Autodesk Inventor part; units mm, degrees
(part 3 of 3)
sketch "Additional Alignment Holes Top" plane through (0, 0, 0) normal (0, 1, 0) x (1, 0, 0)
  circle A0 centre (-38.1, 76.2) radius 3.175 projected
  circle A1 centre (-33.096, 76.2) radius 1.0125 projected
  circle A2 centre (-43.104, 76.2) radius 1.0125 projected
  line L0 (-38.1, 76.2) -> (-38.1, 70.15)
  circle A3 centre (-38.1, 70.15) radius 3.175
  line L1 (-38.1, 70.15) -> (-33.096, 70.15)
  line L2 (-38.1, 70.15) -> (-43.104, 70.15)
  circle A4 centre (-43.104, 70.15) radius 1.0125
  circle A5 centre (-33.096, 70.15) radius 1.0125
  circle A6 centre (-329.6666, 527.8374) radius 3.175 projected
  line L3 (-329.6666, 527.8374) -> (-348.7166, 527.8374)
  circle A7 centre (-348.7166, 527.8374) radius 3.175
  circle A8 centre (-329.6666, 522.8334) radius 1.0125 projected
  circle A9 centre (-329.6666, 532.8414) radius 1.0125 projected
  line L4 (-348.7166, 527.8374) -> (-348.7166, 532.8414)
  line L5 (-348.7166, 527.8374) -> (-348.7166, 522.8334)
  circle A10 centre (-348.7166, 522.8334) radius 1.0125
  circle A11 centre (-348.7166, 532.8414) radius 1.0125
  circle A12 centre (-430.0666, 527.8374) radius 3.175 projected
  line L6 (-430.0666, 527.8374) -> (-404.6666, 527.8374)
  circle A13 centre (-404.6666, 527.8374) radius 3.175
  line L7 (-404.6666, 527.8374) -> (-404.6666, 532.8414)
  circle A14 centre (-404.6666, 522.8334) radius 1.0125
  circle A15 centre (-404.6666, 532.8414) radius 1.0125
  circle A16 centre (-266.1666, 527.8374) radius 3.175 projected
  line L8 (-266.1666, 527.8374) -> (-240.7666, 527.8374)
  circle A17 centre (-240.7666, 527.8374) radius 3.175
  circle A18 centre (-240.7666, 522.8334) radius 1.0125
  circle A19 centre (-240.7666, 532.8414) radius 1.0125
  line L9 (-240.7666, 527.8374) -> (-113.7666, 527.8374)
  circle A20 centre (-113.7666, 527.8374) radius 3.175
  circle A21 centre (-113.7666, 522.8334) radius 1.0125
  circle A22 centre (-113.7666, 532.8414) radius 1.0125
  line L10 (-348.7166, 527.8374) -> (-323.3166, 527.8374)
  line L11 (-323.3166, 527.8374) -> (-323.3166, 502.4374)
  line L12 (-323.3166, 527.8374) -> (-323.3166, 553.2374)
  line L13 (-323.3166, 553.2374) -> (-374.1166, 553.2374)
  line L14 (-374.1166, 553.2374) -> (-374.1166, 502.4374)
  point P0 (0, 0)
  dimension "d807" = 6.05
  dimension "d808" = 6.35
  dimension "d809" = 2.025
  dimension "d810" = 2.025
  dimension "d811" = 19.05
  dimension "d812" = 6.35
  dimension "d813" = 2.025
  dimension "d814" = 2.025
  dimension "d815" = 25.4
  dimension "d816" = 6.35
  dimension "d817" = 2.025
  dimension "d818" = 2.025
  dimension "d819" = 25.4
  dimension "d820" = 6.35
  dimension "d821" = 2.025
  dimension "d822" = 2.025
  dimension "d823" = 127
  dimension "d824" = 6.35
  dimension "d825" = 2.025
  dimension "d826" = 2.025
  dimension "d827" = 25.4
  dimension "d828" = 25.4
  dimension "d829" = 25.4
  dimension "d830" = 50.8
  dimension "d831" = 50.8
  constraints: 30 end point, 15 centre point, 12 coincident, 6 horizontal, 5 vertical, 3 perpendicular, 1 point on line
  measures "d807" distance of L0.start L0.end
  measures "d808" diameter of A3
  measures "d809" diameter of A4
  measures "d810" diameter of A5
  measures "d811" distance of L3.start L3.end
  measures "d812" diameter of A7
  measures "d813" diameter of A10
  measures "d814" diameter of A11
  measures "d815" distance of L6.start L6.end
  measures "d816" diameter of A13
  measures "d817" diameter of A14
  measures "d818" diameter of A15
  measures "d819" distance of L8.start L8.end
  measures "d820" diameter of A17
  measures "d821" diameter of A18
  measures "d822" diameter of A19
  measures "d823" distance of L9.start L9.end
  measures "d824" diameter of A20
  measures "d825" diameter of A21
  measures "d826" diameter of A22
  measures "d827" distance of L4.start L10.end
  measures "d828" distance of L10.end L11.end
  measures "d829" distance of L10.end L12.end
  measures "d830" distance of L12.end L13.end
  measures "d831" distance of L13.end L14.end
hole "Hole4" at (-323.3166, 0, -502.4374) at (-323.3166, 0, -553.2374) at (-374.1166, 0, -553.2374) at (-374.1166, 0, -502.4374) direction (0, -1, 0) diameter 4.9784 end through all thread size "1/4-20 UNC" class "2B" standard "ANSI Unified Screw Threads"
extrude "Extrusion23" cut sketch "Additional Alignment Holes Top" against normal blind 25.4 contours A3 L0 A0 | A0 L0 L2 A3 | A3 L1 L0 A0 | A0 L0 A3 | L2 L1 A3 | A7 L5 L3 | L3 L4 A7 | L5 A7 L4 | A13 L7 L6 | L6 L7 A13 | A17 L9 L8 | L8 L9 A17 | A20
extrude "Extrusion24" cut sketch "Additional Alignment Holes Top" against normal blind 4.445 contours A4 | A5 | A10 | A11 | A14 | A15 | A18 | A19 | A21 | A22
sketch "Sketch26" plane through (-323.3166, -12.7, 0) normal (0, -1, 0) x (1, 0, 0)
  arc A0 (287.8819, -71.8753) -> (282.5513, -71.8753) centre (285.2166, -70.15) ccw projected
  arc A1 (286.181, -73.175) -> (287.8819, -71.8753) centre (285.2166, -70.15) ccw projected
  circle A2 centre (285.2166, -70.15) radius 3.175 projected
  arc A3 (282.5513, -71.8753) -> (287.8819, -71.8753) centre (285.2166, -76.2) ccw projected
  circle A4 centre (285.2166, -70.15) radius 2.54
  circle A5 centre (285.2166, -12.7) radius 5.08 projected
  circle A6 centre (285.2166, -70.15) radius 5.08
  circle A7 centre (209.55, -527.8374) radius 3.175 projected
  circle A8 centre (82.55, -527.8374) radius 3.175 projected
  circle A9 centre (-25.4, -527.8374) radius 3.175 projected
  circle A10 centre (-81.35, -527.8374) radius 3.175 projected
  circle A11 centre (-81.35, -527.8374) radius 5.08
  circle A12 centre (-25.4, -527.8374) radius 5.08
  circle A13 centre (82.55, -527.8374) radius 5.08
  circle A14 centre (209.55, -527.8374) radius 5.08
  point P0 (323.3166, 0)
  dimension "d844" = 10.16
  dimension "d845" = 10.16
  dimension "d846" = 10.16
  dimension "d847" = 10.16
  dimension "d848" = 10.16
  constraints: 6 centre point, 6 coincident
  measures "d844" diameter of A6
  measures "d845" diameter of A11
  measures "d846" diameter of A12
  measures "d847" diameter of A13
  measures "d848" diameter of A14
extrude "Extrusion25" cut sketch "Sketch26" against normal blind 7.62 contours A1 A2 A0 | A3 A6 A2 A1 | A0 A3 A6 | A4 | A7 | A8 | A9 | A10 | A11 | A12 | A13 | A14
sketch "Sketch27" plane through (0, 0, 0) normal (0, 1, 0) x (1, 0, 0)
  arc A0 (-39.0644, 73.175) -> (-37.1356, 73.175) centre (-38.1, 70.15) ccw projected
  arc A1 (-37.1356, 73.175) -> (-39.0644, 73.175) centre (-38.1, 76.2) ccw projected
  line L0 (-38.1, 76.2) -> (-38.1, 63.5)
  circle A2 centre (-38.1, 63.5) radius 3.175
  line L1 (-38.1, 76.2) -> (-38.1, 88.9)
  circle A3 centre (-38.1, 88.9) radius 3.175
  line L2 (-38.1, 76.2) -> (-25.4, 76.2)
  line L3 (-38.1, 76.2) -> (-50.8, 76.2)
  circle A4 centre (-50.8, 76.2) radius 3.175
  circle A5 centre (-25.4, 76.2) radius 3.175
  line L4 (-38.1, 76.2) -> (-16.1, 76.2)
  line L5 (-38.1, 76.2) -> (-38.1, 98.2)
  line L6 (-38.1, 76.2) -> (-38.1, 54.2)
  circle A6 centre (-38.1, 98.2) radius 1.5125
  circle A7 centre (-38.1, 54.2) radius 1.5125
  point P0 (0, 0)
  dimension "d853" = 12.7
  dimension "d854" = 6.35
  dimension "d855" = 12.7
  dimension "d856" = 12.7
  dimension "d857" = 12.7
  dimension "d858" = 6.35
  dimension "d859" = 6.35
  dimension "d860" = 22
  dimension "d861" = 22
  dimension "d862" = 22
  dimension "d863" = 3.025
  dimension "d864" = 3.025
  constraints: 14 end point, 6 centre point, 6 coincident, 3 vertical, 2 horizontal, 1 point on line
  measures "d853" distance of L0.start L0.end
  measures "d854" diameter of A2
  measures "d855" distance of L0.start L1.end
  measures "d856" distance of L0.start L2.end
  measures "d857" distance of L0.start L3.end
  measures "d858" diameter of A4
  measures "d859" diameter of A5
  measures "d860" distance of L0.start L4.end
  measures "d861" distance of L0.start L5.end
  measures "d862" distance of L0.start L6.end
  measures "d863" diameter of A6
  measures "d864" diameter of A7
extrude "Extrusion26" cut sketch "Sketch27" against normal blind 25.4 contours A5 L4 L2 | L2 L4 A5 | A4
extrude "Extrusion27" cut sketch "Sketch27" against normal blind 4.445 contours A6 | A7
sketch "Sketch28" plane through (-323.3166, -12.7, 0) normal (0, -1, 0) x (1, 0, 0)
  circle A0 centre (297.9166, -76.2) radius 3.175 projected
  circle A1 centre (272.5166, -76.2) radius 3.175 projected
  circle A2 centre (297.9166, -76.2) radius 5.08
  circle A3 centre (272.5166, -76.2) radius 5.08
  point P0 (323.3166, 0)
  dimension "d869" = 10.16
  dimension "d870" = 10.16
  constraints: 2 centre point, 2 coincident
  measures "d869" diameter of A2
  measures "d870" diameter of A3
extrude "Extrusion28" cut sketch "Sketch28" against normal blind 7.62 contours A0 | A1 | A2 | A3
hole "Hole5" at (-38.1, 0, -88.9) at (-38.1, 0, -63.5) direction (0, -1, 0) diameter 4.9784 end through all thread size "1/4-20 UNC" class "2B" standard "ANSI Unified Screw Threads"
sketch "Sketch29" plane through (0, 0, 0) normal (0, 1, 0) x (1, 0, 0)
  circle A0 centre (-38.1, 63.5) radius 2.4892 projected
  circle A1 centre (-38.1, 88.9) radius 2.4892 projected
  circle A2 centre (-38.1, 98.2) radius 1.5125 projected
  circle A3 centre (-38.1, 54.2) radius 1.5125 projected
  circle A4 centre (-25.4, 76.2) radius 3.175 projected
  circle A5 centre (-50.8, 76.2) radius 3.175 projected
  circle A6 centre (-113.7666, 532.8414) radius 1.0125 projected
  circle A7 centre (-348.7166, 532.8414) radius 1.0125 projected
  circle A8 centre (-404.6666, 532.8414) radius 1.0125 projected
  circle A9 centre (-240.7666, 532.8414) radius 1.0125 projected
  circle A10 centre (-33.096, 70.15) radius 1.0125 projected
  circle A11 centre (-113.7666, 522.8334) radius 1.0125 projected
  circle A12 centre (-348.7166, 522.8334) radius 1.0125 projected
  circle A13 centre (-404.6666, 522.8334) radius 1.0125 projected
  circle A14 centre (-240.7666, 522.8334) radius 1.0125 projected
  circle A15 centre (-43.104, 70.15) radius 1.0125 projected
  circle A16 centre (-348.7166, 379.0684) radius 3.175 projected
  circle A17 centre (-348.7166, 127.6824) radius 3.175 projected
  circle A18 centre (-348.7166, -46.5176) radius 3.175 projected
  line L0 (-323.3166, 0) -> (0, 0) projected
  line L1 (0, 0) -> (0, 565.9374) projected
  line L2 (0, 565.9374) -> (-329.6666, 565.9374) projected
  line L3 (-329.6666, 565.9374) -> (-329.6666, 604.0374) projected
  line L4 (-329.6666, 604.0374) -> (-367.7666, 604.0374) projected
  line L5 (-367.7666, 604.0374) -> (-367.7666, 565.9374) projected
  line L6 (-367.7666, 565.9374) -> (-705.4595, 565.9374) projected
  line L7 (-705.4595, 565.9374) -> (-705.4595, 489.7374) projected
  line L8 (-705.4595, 489.7374) -> (-374.1166, 489.7374) projected
  line L9 (-374.1166, 489.7374) -> (-374.1166, -84.6176) projected
  line L10 (-374.1166, -84.6176) -> (-323.3166, -84.6176) projected
  line L11 (-323.3166, -84.6176) -> (-323.3166, 0) projected
  circle A19 centre (-266.1666, 527.8374) radius 3.175 projected
  circle A20 centre (-88.9, 489.7374) radius 3.175 projected
  circle A21 centre (-38.1, 338.92) radius 3.175 projected
  circle A22 centre (-38.1, 12.7) radius 3.175 projected
  arc A23 (-39.0644, 73.175) -> (-37.1356, 73.175) centre (-38.1, 70.15) ccw projected
  arc A24 (-37.1356, 73.175) -> (-39.0644, 73.175) centre (-38.1, 76.2) ccw projected
  circle A25 centre (-38.1, 156.845) radius 3.175 projected
  circle A26 centre (-38.1, 173.736) radius 3.175 projected
  circle A27 centre (-38.1, 243.84) radius 3.175 projected
  circle A28 centre (-26.0664, 539.871) radius 3.175 projected
  circle A29 centre (-38.1, 424.2816) radius 3.175 projected
  circle A30 centre (-329.6666, 527.8374) radius 3.175 projected
  circle A31 centre (-431.1336, 515.8038) radius 3.175 projected
  circle A32 centre (-419.1, 553.2374) radius 3.175 projected
  circle A33 centre (-494.6675, 527.8374) radius 3.175 projected
  circle A34 centre (-329.6666, 522.8334) radius 1.0125 projected
  circle A35 centre (-29.6048, 543.4093) radius 1.0125 projected
  circle A36 centre (-434.6719, 519.3422) radius 1.0125 projected
  circle A37 centre (-494.6675, 522.8334) radius 1.0125 projected
  circle A38 centre (-43.104, 76.2) radius 1.0125 projected
  circle A39 centre (-43.104, 173.736) radius 1.0125 projected
  circle A40 centre (-43.104, 424.2816) radius 1.0125 projected
  circle A41 centre (-93.904, 489.7374) radius 1.0125 projected
  circle A42 centre (-33.096, 243.84) radius 1.0125 projected
  circle A43 centre (-33.096, 156.845) radius 1.0125 projected
  circle A44 centre (-43.104, 12.7) radius 1.0125 projected
  circle A45 centre (-414.096, 553.2374) radius 1.0125 projected
  circle A46 centre (-266.1666, 532.8414) radius 1.0125 projected
  circle A47 centre (-33.096, 338.92) radius 1.0125 projected
  circle A48 centre (-329.6666, 532.8414) radius 1.0125 projected
  circle A49 centre (-22.5281, 536.3326) radius 1.0125 projected
  circle A50 centre (-427.5952, 512.2655) radius 1.0125 projected
  circle A51 centre (-494.6675, 532.8414) radius 1.0125 projected
  circle A52 centre (-33.096, 76.2) radius 1.0125 projected
  circle A53 centre (-33.096, 173.736) radius 1.0125 projected
  circle A54 centre (-33.096, 424.2816) radius 1.0125 projected
  circle A55 centre (-83.896, 489.7374) radius 1.0125 projected
  circle A56 centre (-43.104, 243.84) radius 1.0125 projected
  circle A57 centre (-43.104, 156.845) radius 1.0125 projected
  circle A58 centre (-33.096, 12.7) radius 1.0125 projected
  circle A59 centre (-424.104, 553.2374) radius 1.0125 projected
  circle A60 centre (-266.1666, 522.8334) radius 1.0125 projected
  circle A61 centre (-43.104, 338.92) radius 1.0125 projected
  circle A62 centre (-353.7206, 379.0684) radius 1.0125 projected
  circle A63 centre (-353.7206, -46.5176) radius 1.0125 projected
  circle A64 centre (-343.7126, 127.6824) radius 1.0125 projected
  circle A65 centre (-343.7126, 379.0684) radius 1.0125 projected
  circle A66 centre (-343.7126, -46.5176) radius 1.0125 projected
  circle A67 centre (-353.7206, 127.6824) radius 1.0125 projected
  circle A68 centre (-639.4195, 502.4374) radius 2.4892 projected
  circle A69 centre (-690.2195, 502.4374) radius 2.4892 projected
  circle A70 centre (-639.4195, 553.2374) radius 2.4892 projected
  circle A71 centre (-12.7, 12.7) radius 5.08 projected
  circle A72 centre (-342.9, 495.3) radius 5.08 projected
  circle A73 centre (-698.5, 546.1) radius 5.08 projected
  circle A74 centre (-114.3, 12.7) radius 5.08 projected
  circle A75 centre (-114.3, 495.3) radius 5.08 projected
  circle A76 centre (-698.5, 495.3) radius 5.08 projected
  circle A77 centre (-342.9, -12.7) radius 5.08 projected
  circle A78 centre (-12.7, 546.1) radius 5.08 projected
  circle A79 centre (-348.7166, 145.8734) radius 3.175 projected
  circle A80 centre (-348.7166, -34.0266) radius 3.175 projected
  circle A81 centre (-343.7126, 145.8734) radius 1.0125 projected
  circle A82 centre (-343.7126, -34.0266) radius 1.0125 projected
  circle A83 centre (-353.7206, 145.8734) radius 1.0125 projected
  circle A84 centre (-353.7206, -34.0266) radius 1.0125 projected
  circle A85 centre (-574.8186, 502.4374) radius 2.4892 projected
  circle A86 centre (-574.8186, 553.2374) radius 2.4892 projected
  circle A87 centre (-625.6186, 502.4374) radius 2.4892 projected
  circle A88 centre (-228.2976, 80.7174) radius 3.175 projected
  circle A89 centre (-228.2976, 282.2874) radius 3.175 projected
  circle A90 centre (-216.264, 539.871) radius 3.175 projected
  circle A91 centre (-348.7166, 138.1034) radius 3.175 projected
  circle A92 centre (-348.7166, 389.0574) radius 3.175 projected
  circle A93 centre (-279.0976, 413.5374) radius 3.175 projected
  circle A94 centre (-228.2976, 244.1874) radius 3.175 projected
  circle A95 centre (-228.2976, 156.9174) radius 3.175 projected
  circle A96 centre (-228.2976, 320.3874) radius 3.175 projected
  circle A97 centre (-291.5666, 527.8374) radius 3.175 projected
  circle A98 centre (-348.7166, -75.3966) radius 3.175 projected
  circle A99 centre (-430.0666, 527.8374) radius 3.175 projected
  circle A100 centre (-228.2976, 409.7056) radius 3.175 projected
  circle A101 centre (-228.2976, 174.0274) radius 3.175 projected
  circle A102 centre (-348.7166, -53.4156) radius 3.175 projected
  circle A103 centre (-348.7166, 156.3064) radius 3.175 projected
  circle A104 centre (-343.7126, 389.0574) radius 1.0125 projected
  circle A105 centre (-343.7126, 138.1034) radius 1.0125 projected
  circle A106 centre (-291.5666, 522.8334) radius 1.0125 projected
  circle A107 centre (-233.3016, 409.7056) radius 1.0125 projected
  circle A108 centre (-223.2936, 320.3874) radius 1.0125 projected
  circle A109 centre (-233.3016, 244.1874) radius 1.0125 projected
  circle A110 centre (-233.3016, 156.9174) radius 1.0125 projected
  circle A111 centre (-223.2936, 80.7174) radius 1.0125 projected
  circle A112 centre (-223.2936, 174.0274) radius 1.0125 projected
  circle A113 centre (-223.2936, 282.2874) radius 1.0125 projected
  circle A114 centre (-284.1016, 413.5374) radius 1.0125 projected
  circle A115 centre (-212.7257, 536.3326) radius 1.0125 projected
  circle A116 centre (-430.0666, 522.8334) radius 1.0125 projected
  circle A117 centre (-353.7206, -75.3966) radius 1.0125 projected
  circle A118 centre (-353.7206, 389.0574) radius 1.0125 projected
  circle A119 centre (-353.7206, 138.1034) radius 1.0125 projected
  circle A120 centre (-291.5666, 532.8414) radius 1.0125 projected
  circle A121 centre (-223.2936, 409.7056) radius 1.0125 projected
  circle A122 centre (-233.3016, 320.3874) radius 1.0125 projected
  circle A123 centre (-223.2936, 244.1874) radius 1.0125 projected
  circle A124 centre (-223.2936, 156.9174) radius 1.0125 projected
  circle A125 centre (-233.3016, 80.7174) radius 1.0125 projected
  circle A126 centre (-233.3016, 174.0274) radius 1.0125 projected
  circle A127 centre (-233.3016, 282.2874) radius 1.0125 projected
  circle A128 centre (-274.0936, 413.5374) radius 1.0125 projected
  circle A129 centre (-219.8024, 543.4093) radius 1.0125 projected
  circle A130 centre (-430.0666, 532.8414) radius 1.0125 projected
  circle A131 centre (-343.7126, -75.3966) radius 1.0125 projected
  circle A132 centre (-353.7206, -53.4156) radius 1.0125 projected
  circle A133 centre (-343.7126, -53.4156) radius 1.0125 projected
  circle A134 centre (-343.7126, 156.3064) radius 1.0125 projected
  circle A135 centre (-353.7206, 156.3064) radius 1.0125 projected
  circle A136 centre (-343.7126, 591.3374) radius 1.0125 projected
  circle A137 centre (-353.7206, 591.3374) radius 1.0125 projected
  circle A138 centre (-348.7166, 591.3374) radius 3.175 projected
  circle A139 centre (-323.3166, 502.4374) radius 2.4892 projected
  circle A140 centre (-323.3166, 553.2374) radius 2.4892 projected
  circle A141 centre (-374.1166, 553.2374) radius 2.4892 projected
  circle A142 centre (-374.1166, 502.4374) radius 2.4892 projected
  circle A143 centre (-113.7666, 527.8374) radius 3.175 projected
  circle A144 centre (-240.7666, 527.8374) radius 3.175 projected
  circle A145 centre (-348.7166, 527.8374) radius 3.175 projected
  circle A146 centre (-404.6666, 527.8374) radius 3.175 projected
body "Solid1"
